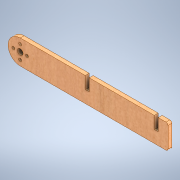
# Autodesk Inventor part: Деталь 3
Saved by Autodesk Inventor 2020.1 (Build 241239000, 239)
## iProperties
Created: 2021-08-12
Part Number: Деталь 3
Material: Дерево (вишня)
Document SubType Name: Modeling
Designer: Ni3na
Density: 0.63 g/cm^3
Appearance: Вишневое дерево — натуральный — со слабым глянцем
Author: Ni3na
Autodesk Inventor part; units mm, degrees
ref_plane "YZ Plane" through (0, 0, 0) normal (1, 0, 0) x (0, 1, 0)
ref_plane "XZ Plane" through (0, 0, 0) normal (0, 1, 0) x (-1, 0, 0)
ref_plane "XY Plane" through (0, 0, 0) normal (0, 0, 1) x (1, 0, 0)
sketch "Эскиз1" plane through (0, 0, 0) normal (0, 0, 1) x (1, 0, 0)
  circle A0 centre (0, 0) radius 12.5
  line L0 (0, -12.5) -> (280, -12.5)
  line L1 (280, -12.5) -> (280, 12.5)
  line L2 (280, 12.5) -> (0, 12.5)
  line L3 (0, 12.5) -> (0, -12.5)
  circle A1 centre (280, 0) radius 12.5
  circle A2 centre (0, 0) radius 7
  circle A3 centre (280, 0) radius 7
  circle A4 centre (0, 7) radius 1.5
  circle A5 centre (7, 0) radius 1.5
  circle A6 centre (0, -7) radius 1.5
  circle A7 centre (-7, 0) radius 1.5
  circle A8 centre (0, 0) radius 3
  circle A9 centre (280, 0) radius 3
  circle A10 centre (287, 0) radius 1.5
  circle A11 centre (280, 7) radius 1.5
  circle A12 centre (280, -7) radius 1.5
  circle A13 centre (273, 0) radius 1.5
  line L4 (138, 12.5) -> (142, 12.5)
  line L5 (142, 12.5) -> (142, 0)
  line L6 (142, 0) -> (138, 0)
  line L7 (138, 0) -> (138, 12.5)
  point P0 (280, -12.5)
  point P1 (140, 12.5)
  point P2 (140, 12.5)
  point P3 (142, 12.5)
  dimension "d0" = 25
  dimension "d2" = 14
  dimension "d3" = 14
  dimension "d4" = 3
  dimension "d5" = 3
  dimension "d6" = 3
  dimension "d7" = 3
  dimension "d8" = 6
  dimension "d9" = 6
  dimension "d10" = 3
  dimension "d11" = 3
  dimension "d12" = 3
  dimension "d13" = 3
  dimension "d16" = 0
  dimension "d17" = 4
  dimension "d27" = 280
  constraints: 16 end point, 12 centre point, 8 point on circle, 5 coincident, 5 point on line, 4 parallel, 3 midpoint, 2 horizontal, 2 perpendicular, 6 other
  measures "d2" diameter of A2
  measures "d3" diameter of A3
  measures "d4" diameter of A4
  measures "d5" diameter of A5
  measures "d6" diameter of A6
  measures "d7" diameter of A7
  measures "d8" diameter of A8
  measures "d9" diameter of A9
  measures "d10" diameter of A10
  measures "d11" diameter of A11
  measures "d12" diameter of A12
  measures "d13" diameter of A13
  measures "d16" distance of point (140, 12.5) point (140, 12.5)
  measures "d17" distance of L5.end L6.end
  measures "d27" distance of point (280, 0) point (0, 0)
extrude "Выдавливание1" add sketch "Эскиз1" along normal blind 4 contours A0 L3 A6 A2 A5 A4 | A0 L2 L7 L6 L5 A1 L0 | L3 A4 A2 A7 A6 A0 | A1 L1 A11 A3 A13 A12 | L1 A12 A3 A10 A11 A1 | A4 L3 A8 A6 A2 A7 | A4 A2 A5 A6 L3 A8 | A3 A13 A11 L1 A9 A12 | L1 A9 A11 A3 A10 A12
sketch "Эскиз2" plane through (0, 0, 4) normal (0, 0, 1) x (1, 0, 0)
  line L0 (152, 23.4347) -> (358.3941, 23.4347)
  line L1 (358.3941, 23.4347) -> (358.3941, -33.9487)
  line L2 (358.3941, -33.9487) -> (152, -33.9487)
  line L3 (152, -33.9487) -> (152, 23.4347)
  line L4 (142, 12.5) -> (142, 0) projected
  point P0 (0, 0)
  dimension "d18" = 10
  constraints: 8 end point, 2 parallel, 1 horizontal, 1 perpendicular
  measures "d18" distance from line of L4 L0.start
extrude "Выдавливание2" cut sketch "Эскиз2" against normal blind 10
fillet "Сопряжение1" radius 2 2 edges at (152, 12.5, 2) (152, -12.5, 2)
sketch "Эскиз3" plane through (0, 0, 4) normal (0, 0, 1) x (1, 0, 0)
  line L0 (138, 12.5) -> (0, 12.5) projected
  line L1 (67, 12.5) -> (71, 12.5)
  line L2 (71, 12.5) -> (71, 0)
  line L3 (71, 0) -> (67, 0)
  line L4 (67, 0) -> (67, 12.5)
  line L5 (142, 0) -> (138, 0) projected
  point P0 (0, 0)
  point P1 (69, 12.5)
  point P2 (69, 12.5)
  point P3 (71, 12.5)
  point P4 (140, 0)
  dimension "d22" = 0
  dimension "d23" = 4
  constraints: 8 end point, 3 midpoint, 2 parallel, 1 horizontal, 1 perpendicular, 1 point on line
  measures "d22" distance of point (69, 12.5) point (69, 12.5)
  measures "d23" distance of L2.end L3.end
extrude "Выдавливание3" cut sketch "Эскиз3" against normal blind 10
